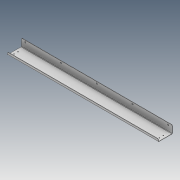
# Autodesk Inventor part: Xaxis_Dragchain_Guide
Saved by Autodesk Inventor 2020 (Build 240168000, 168)
## iProperties
Created: 2020-11-10
Part Number: Xaxis_Dragchain_Guide
Material: Generic
Document SubType Name: Sheet Metal
Designer: magnarecta
Density: 1 g/cm^3
Sheet Metal Rule: Default_mm
Appearance: Default
Author: magnarecta
Autodesk Inventor part; units mm, degrees
ref_plane "YZ Plane" through (0, 0, 0) normal (1, 0, 0) x (0, 1, 0)
ref_plane "XZ Plane" through (0, 0, 0) normal (0, 1, 0) x (-1, 0, 0)
sketch "Sketch1" plane through (0, 0, 0) normal (0, 0, 1) x (1, 0, 0)
  line L0 (290, -15) -> (-290, -15)
  line L1 (-290, -15) -> (-290, 15)
  line L2 (-290, 15) -> (290, 15)
  line L3 (290, 15) -> (290, -15)
  line L4 (290, -15) -> (-290, 15) construction
  line L5 (-290, -15) -> (290, 15) construction
  point P0 (0, 0)
  dimension "d0" = 580
  dimension "d1" = 30
  measures "d0" distance of L1.end L2.end
  measures "d1" distance of L0.end L1.end
extrude "Plate1" add sketch "Sketch1" along normal blind 1.5
sketch "Sketch2" plane through (290, -13.5, 0) normal (0, -1, 0) x (1, 0, 0)
  line L0 (-580, 0) -> (0, 0)
  line L1 (0, 0) -> (0, 55)
  line L2 (0, 55) -> (-580, 55)
  line L3 (-580, 55) -> (-580, 0)
  constraints: 6 end point, 1 horizontal, 1 perpendicular, 1 vertical
edge flange "Flange1" height 55 angle 90 thickness 1.5 bend radius 1.5 thickness toward (0, -1, 0) relief tear relief width 1.5 relief depth 0.75 edges at (0, -15, 1.5) wall of the first edge with corners at (-290, -13.5, 0) (290, -13.5, 0) (290, -13.5, 55) (-290, -13.5, 55)
bend "Bend1"
corner "Corner1"
sketch "Sketch3" plane through (290, -15, 53.5) normal (0, 0, 1) x (1, 0, 0)
  line L0 (-580, 0) -> (0, 0)
  line L1 (0, 0) -> (0, 10)
  line L2 (0, 10) -> (-580, 10)
  line L3 (-580, 10) -> (-580, 0)
  constraints: 6 end point, 1 horizontal, 1 perpendicular, 1 vertical
edge flange "Flange2" height 10 angle 90 thickness 1.5 bend radius 1.5 thickness toward (0, 0, 1) relief tear relief width 1.5 relief depth 0.75 edges at (0, -13.5, 55) wall of the first edge with corners at (-290, -15, 53.5) (290, -15, 53.5) (290, -5, 53.5) (-290, -5, 53.5)
bend "Bend2"
corner "Corner2"
sketch "スケッチ4" plane through (0, 0, 1.5) normal (0, 0, 1) x (1, 0, 0)
  line L0 (-290, -12) -> (290, -12) projected
  line L1 (290, 15) -> (290, -12) projected
  line L2 (-290, 15) -> (290, 15) projected
  line L3 (-290, -12) -> (-290, 15) projected
  point P0 (0, 0)
  point P1 (-275, 8.5)
  point P2 (275, 8.5)
  point P3 (0, 8.5)
  point P4 (-137.5, 8.5)
  point P5 (137.5, 8.5)
  dimension "d24" = 15
  dimension "d25" = 15
  dimension "d27" = 137.5
  dimension "d58" = 137.5
  dimension "d59" = 275
  constraints: 3 horizontal alignment, 1 vertical alignment
  measures "d24" distance from line of point (-275, 8.5) L3
  measures "d25" distance from line of point (275, 8.5) L1
  measures "d27" distance of point (0, 8.5) point (-137.5, 8.5)
  measures "d58" distance of point (137.5, 8.5) point (0, 8.5)
  measures "d59" distance of point (0, 8.5) point (-275, 8.5)
hole "穴1" at (-275, 8.5, 1.5) at (275, 8.5, 1.5) at (0, 8.5, 1.5) at (-137.5, 8.5, 1.5) at (137.5, 8.5, 1.5) direction (0, 0, -1) diameter 5.2 depth 1.5 tip angle 118
fillet "フィレット1" radius 3 4 edges at (290, -5, 54.25) (290, 15, 0.75) (-290, -5, 54.25) (-290, 15, 0.75)
sketch "スケッチ5" plane through (-290, -13.5, 3) normal (0, 1, 0) x (1, 0, 0)
  line L0 (0, -49) -> (580, -49) projected
  line L1 (580, 0) -> (580, -49) projected
  line L2 (580, 0) -> (0, 0) projected
  line L3 (0, 0) -> (0, -49) projected
  line L4 (0, 0) -> (0, -49) projected
  point P0 (290, 3)
  point P1 (10, -37)
  point P2 (10, -22)
  point P3 (10, -29.5)
  dimension "d36" = 15
  dimension "d40" = 10
  dimension "d60" = 7.5
  dimension "d61" = 19.5
  constraints: 2 vertical alignment
  measures "d36" distance of point (10, -22) point (10, -37)
  measures "d40" distance from line of point (10, -37) L3
  measures "d60" distance of point (10, -22) point (10, -29.5)
  measures "d61" distance from line of point (10, -29.5) L0
hole "穴2" at (-280, -13.5, 40) at (-280, -13.5, 25) direction (0, -1, 0) diameter 3.242 end through all thread size "M4x0.7" class "6H" standard "ISO Metric profile"
ref_plane "作業平面1" through (-45, -12, 1.5) normal (1, 0, 0) x (0, 0, -1)
sketch "Sketch7" plane through (-290, -13.5, 3) normal (0, 1, 0) x (1, 0, 0)
  circle A0 centre (10, -37) radius 1.621 projected
  circle A1 centre (10, -22) radius 1.621 projected
  line L0 (0, -49) -> (580, -49) projected
  line L1 (580, 0) -> (580, -49) projected
  line L2 (580, 0) -> (0, 0) projected
  line L3 (0, 0) -> (0, -49) projected
  point P0 (290, 3)
  point P1 (570, -22)
  point P2 (570, -37)
  dimension "d50" = 10
  constraints: 2 horizontal alignment, 1 vertical alignment
  measures "d50" distance from line of L1 point (570, -22)
hole "Hole3" at (280, -13.5, 25) at (280, -13.5, 40) direction (0, -1, 0) diameter 3.242 end through all thread size "M4x0.7" class "6H" standard "ISO Metric profile"
equation "\"d27\" = 0.5 * d59"
equation "\"d58\" = 0.5 * d59"
equation "\"d33\" = Thickness"
equation "\"d2\" = Thickness"
equation "\"d3\" = BendReliefWidth"
equation "\"d4\" = BendReliefDepth"
equation "\"d5\" = MinimumRemnant"
equation "\"d6\" = TransitionRadius"
equation "\"d9\" = BendRadius"
equation "\"d10\" = CornerReliefSize"
equation "\"d11\" = GapSize"
equation "\"d12\" = JacobiRadiusSize"
equation "\"d13\" = BendReliefWidth"
equation "\"d14\" = BendReliefDepth"
equation "\"d15\" = MinimumRemnant"
equation "\"d16\" = TransitionRadius"
equation "\"d19\" = BendRadius"
equation "\"d20\" = CornerReliefSize"
equation "\"d21\" = GapSize"
equation "\"d22\" = JacobiRadiusSize"
equation "\"BendRadius\" = Thickness"
equation "\"BendReliefWidth\" = Thickness"
equation "\"BendReliefDepth\" = 0.5 * Thickness"
equation "\"CornerReliefSize\" = 4 * Thickness"
equation "\"MinimumRemnant\" = 2 * Thickness"
equation "\"TransitionRadius\" = BendRadius"
equation "\"JacobiRadiusSize\" = BendRadius"
equation "\"GapSize\" = Thickness"
equation "\"Thickness\" = 1.5"
body "Solid1"
